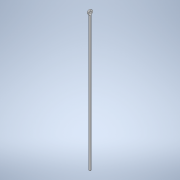
# Autodesk Inventor part: guide
Saved by Autodesk Inventor 2020 (Build 240168000, 168)
## iProperties
Created: 2020-05-22
Part Number: guide
Material: Generic
Document SubType Name: Modeling
Designer: alejandrosalazar
Density: 1 g/cm^3
Appearance: Default
Author: alejandrosalazar
Autodesk Inventor part; units mm, degrees
ref_plane "YZ Plane" through (0, 0, 0) normal (1, 0, 0) x (0, 1, 0)
ref_plane "XZ Plane" through (0, 0, 0) normal (0, 1, 0) x (-1, 0, 0)
ref_plane "XY Plane" through (0, 0, 0) normal (0, 0, 1) x (1, 0, 0)
sketch "Sketch4" plane through (0, 0, 0) normal (1, 0, 0) x (0, 1, 0)
  line L0 (0, 0) -> (280, 0)
  line L1 (280, 0) -> (280, -2)
  line L2 (280, -2) -> (0, -2)
  line L3 (0, -2) -> (0, 0)
  circle A0 centre (282.55, -1) radius 2.625
  circle A1 centre (282.55, -1) radius 4.5
  point P0 (278.1625, -2)
  point P1 (278.1625, 0)
  dimension "d10" = 280
  dimension "d11" = 2
  dimension "d12" = 5.25
  dimension "d13" = 9
  constraints: 8 end point, 2 centre point, 2 parallel, 1 coincident, 1 horizontal, 1 perpendicular
  measures "d10" distance of L1.end L2.end
  measures "d11" distance of L0.end L1.end
  measures "d12" diameter of A0
  measures "d13" diameter of A1
extrude "Extrusion2" add sketch "Sketch4" along normal blind 2.4 contours L0 A1 L2 L3 | A1 L2 L1 A0 L0 | L0 L1 A0 L2 A1
sketch "Sketch6" plane through (0, 0, -2) normal (0, -1, 0) x (1, 0, 0)
  line L0 (0, 2) -> (0, 0) projected
  line L1 (0, 0) -> (2.4, 0)
  line L2 (2.4, 0) -> (2.4, 2)
  line L3 (2.4, 2) -> (0, 2)
  line L4 (0, 2) -> (0, 0)
  constraints: 8 end point, 2 parallel, 1 horizontal, 1 perpendicular
extrude "Extrusion4" add sketch "Sketch6" along normal blind 5
body "Solid2"
